hex_lightcovertest (Autodesk Fusion 360 design; units mm, degrees)
Autodesk Fusion 360 part; units mm, degrees
sketch "Sketch1" plane through (0, 12, 0) normal (0, -1, 0) x (1, 0, 0)
  line L0 (-41.8393, 72.4678) -> (-83.6786, 0)
  line L1 (-83.6786, 0) -> (-41.8393, -72.4678)
  line L2 (-41.8393, -72.4678) -> (41.8393, -72.4678)
  line L3 (41.8393, -72.4678) -> (83.6786, 0)
  line L4 (83.6786, 0) -> (41.8393, 72.4678)
  line L5 (41.8393, 72.4678) -> (-41.8393, 72.4678)
  line L6 (-41.8393, 72.4678) -> (41.8393, 72.4678)
  line L7 (41.8393, 72.4678) -> (83.6786, 0)
  line L8 (83.6786, 0) -> (41.8393, -72.4678)
  line L9 (41.8393, -72.4678) -> (-41.8393, -72.4678)
  line L10 (-41.8393, -72.4678) -> (-83.6786, 0)
  line L11 (-83.6786, 0) -> (-41.8393, 72.4678)
  line L12 (82.0621, 0) -> (41.031, -71.0678)
  line L13 (41.031, -71.0678) -> (-41.031, -71.0678)
  line L14 (-41.031, -71.0678) -> (-82.0621, 0)
  line L15 (-82.0621, 0) -> (-41.031, 71.0678)
  line L16 (-41.031, 71.0678) -> (41.031, 71.0678)
  line L17 (41.031, 71.0678) -> (82.0621, 0)
  dimension "d1" = 1.4
  constraint coincident L0.start L5.end
  constraint coincident L4.end L5.start
  constraint coincident L3.end L4.start
  constraint coincident L2.end L3.start
  constraint coincident L1.end L2.start
  constraint coincident L0.end L1.start
sketch "Sketch2" plane through (0, 12, 0) normal (0, 1, 0) x (-1, 0, 0)
  line L0 (-42.4167, 73.4678) -> (42.4167, 73.4678)
  line L1 (42.4167, 73.4678) -> (84.8333, 0)
  line L2 (84.8333, 0) -> (42.4167, -73.4678)
  line L3 (42.4167, -73.4678) -> (-42.4167, -73.4678)
  line L4 (-42.4167, -73.4678) -> (-84.8333, 0)
  line L5 (-84.8333, 0) -> (-42.4167, 73.4678)
  line L6 (-43.5714, 75.4678) -> (-87.1427, 0)
  line L7 (-87.1427, 0) -> (-43.5714, -75.4678)
  line L8 (-43.5714, -75.4678) -> (43.5714, -75.4678)
  line L9 (43.5714, -75.4678) -> (87.1427, 0)
  line L10 (87.1427, 0) -> (43.5714, 75.4678)
  line L11 (43.5714, 75.4678) -> (-43.5714, 75.4678)
  line L12 (-43.5714, 75.4678) -> (43.5714, 75.4678)
  line L13 (87.1427, 0) -> (43.5714, 75.4678)
  line L14 (87.1427, 0) -> (43.5714, -75.4678)
  line L15 (43.5714, -75.4678) -> (-43.5714, -75.4678)
  line L16 (-43.5714, -75.4678) -> (-87.1427, 0)
  line L17 (-87.1427, 0) -> (-43.5714, 75.4678)
  constraint coincident L6.start L11.end
  constraint coincident L10.end L11.start
  constraint coincident L9.end L10.start
  constraint coincident L8.end L9.start
  constraint coincident L7.end L8.start
  constraint coincident L6.end L7.start
sketch "Sketch3" plane through (0, 4, 0) normal (0, 1, 0) x (-1, 0, 0)
  line L0 (-38.9526, -67.4678) -> (-77.9051, 0)
  line L1 (-77.9051, 0) -> (-38.9526, 67.4678)
  line L2 (-38.9526, 67.4678) -> (38.9526, 67.4678)
  line L3 (38.9526, 67.4678) -> (77.9051, 0)
  line L4 (77.9051, 0) -> (38.9526, -67.4678)
  line L5 (38.9526, -67.4678) -> (-38.9526, -67.4678)
  line L6 (-84.8333, 0) -> (-42.4167, -73.4678)
  line L7 (-42.4167, -73.4678) -> (42.4167, -73.4678)
  line L8 (42.4167, -73.4678) -> (84.8333, 0)
  line L9 (84.8333, 0) -> (42.4167, 73.4678)
  line L10 (42.4167, 73.4678) -> (-42.4167, 73.4678)
  line L11 (-42.4167, 73.4678) -> (-84.8333, 0)
  line L12 (42.4167, -73.4678) -> (84.8333, 0)
  line L13 (42.4167, 73.4678) -> (84.8333, 0)
  line L14 (42.4167, 73.4678) -> (-42.4167, 73.4678)
  line L15 (-42.4167, 73.4678) -> (-84.8333, 0)
  line L16 (-84.8333, 0) -> (-42.4167, -73.4678)
  line L17 (-42.4167, -73.4678) -> (42.4167, -73.4678)
  line L18 (-42.4167, 73.4678) -> (-84.8333, 0)
  line L19 (-41.8393, -72.4678) -> (41.8393, -72.4678)
  line L20 (41.8393, -72.4678) -> (83.6786, 0)
  line L21 (41.8393, 72.4678) -> (83.6786, 0)
  line L22 (41.8393, 72.4678) -> (-41.8393, 72.4678)
  line L23 (-41.8393, 72.4678) -> (-83.6786, 0)
  line L24 (-83.6786, 0) -> (-41.8393, -72.4678)
  line L25 (41.031, 71.0678) -> (-41.031, 71.0678)
  line L26 (-41.031, 71.0678) -> (-82.0621, 0)
  line L27 (-82.0621, 0) -> (-41.031, -71.0678)
  line L28 (-41.031, -71.0678) -> (41.031, -71.0678)
  line L29 (41.031, -71.0678) -> (82.0621, 0)
  line L30 (41.031, 71.0678) -> (82.0621, 0)
  dimension "d2" = -1
  dimension "d3" = -2.4
  constraint coincident L7.end L8.start
  constraint coincident L8.end L9.start
  constraint coincident L9.end L10.start
  constraint coincident L10.end L11.start
  constraint coincident L6.start L11.end
  constraint coincident L6.end L7.start
sketch "Sketch4" plane through (0, 13, 0) normal (0, -1, 0) x (1, 0, 0)
  arc A0 (44.7261, 67.4678) -> (36.0658, 72.4678) centre (36.0658, 62.4678) ccw
  line L0 (44.7261, 67.4678) -> (80.7919, 5)
  arc A1 (80.7919, -5) -> (80.7919, 5) centre (72.1316, 0) ccw
  line L1 (80.7919, -5) -> (44.7261, -67.4678)
  arc A2 (36.0658, -72.4678) -> (44.7261, -67.4678) centre (36.0658, -62.4678) ccw
  line L2 (36.0658, -72.4678) -> (-36.0658, -72.4678)
  arc A3 (-44.7261, -67.4678) -> (-36.0658, -72.4678) centre (-36.0658, -62.4678) ccw
  line L3 (-44.7261, -67.4678) -> (-80.7919, -5)
  arc A4 (-80.7919, 5) -> (-80.7919, -5) centre (-72.1316, 0) ccw
  line L4 (-80.7919, 5) -> (-44.7261, 67.4678)
  arc A5 (-36.0658, 72.4678) -> (-44.7261, 67.4678) centre (-36.0658, 62.4678) ccw
  line L5 (-36.0658, 72.4678) -> (36.0658, 72.4678)
  line L6 (42.4167, 73.4678) -> (-42.4167, 73.4678)
  line L7 (-42.4167, 73.4678) -> (-84.8333, 0)
  line L8 (-84.8333, 0) -> (-42.4167, -73.4678)
  line L9 (-42.4167, -73.4678) -> (42.4167, -73.4678)
  line L10 (42.4167, -73.4678) -> (84.8333, 0)
  line L11 (84.8333, 0) -> (42.4167, 73.4678)
  line L12 (-42.4167, 73.4678) -> (-32.4167, 73.4678)
  line L13 (-42.4167, 73.4678) -> (-47.4167, 64.8076)
  line L14 (-32.4167, 73.4678) -> (-32.4167, 56.1473)
  line L15 (-47.4167, 64.8076) -> (-32.4167, 56.1473)
  dimension "d4" = 10
  dimension "d5" = 0
  constraint coincident L6.end L7.start
  constraint coincident L6 L12.end
  constraint parallel L6 L12
  constraint coincident L7 L13.end
  constraint parallel L7 L13
  constraint perpendicular L5 L14
  constraint perpendicular L13 L15
  constraint coincident L14.end L15.end
  measures "d4" distance of L6.end L13.end
  measures "d5" distance of L6.end L12.end
extrude "Extrude1" add sketch "Sketch2" along normal blind 3 contours L0 L1 L2 L3 L4 L5 | L6 L7 L8 L9 L10 L11 L12 L13 L14 L15 L16 L17
extrude "Extrude2" cut sketch "Sketch3" along normal blind -1 and the other way blind -9 contours L6 L7 L8 L9 L10 L11 L12 L13 L14 L15 L16 L17 L18
move_face "OffsetFaces1" [suppressed]
extrude "Extrude3" cut sketch "Sketch1" against normal blind 2.6 contours L12 L13 L14 L15 L16 L17
fillet "Fillet1" radius 10 6 edges at (-83.6786, 12.5, 0) (-41.8393, 12.5, 72.4678) (41.8393, 12.5, 72.4678) (83.6786, 12.5, 0) (41.8393, 12.5, -72.4678) (-41.8393, 12.5, -72.4678)
fillet "Fillet1" radius 10 6 edges at (-41.031, 13.3, 71.0678) (-82.0621, 13.3, 0) (-41.031, 13.3, -71.0678) (41.031, 13.3, -71.0678) (82.0621, 13.3, 0) (41.031, 13.3, 71.0678)
chamfer "Chamfer1" distance 1 angle 45 18 edges at (63.625, 12, 36.7339) (63.625, 12, -36.7339) (82.1316, 12, 0) (62.759, 12, -36.2339) (41.0658, 12, -71.1281) (0, 12, -72.4678) (-41.0658, 12, -71.1281) (-62.759, 12, -36.2339) (-82.1316, 12, 0) (-62.759, 12, 36.2339) (-41.0658, 12, 71.1281) (0, 12, 72.4678) (41.0658, 12, 71.1281) (62.759, 12, 36.2339) (0, 12, 73.4678) (-63.625, 12, 36.7339) (-63.625, 12, -36.7339) (0, 12, -73.4678)
sketch "Sketch5" plane through (0, 14.6, 0) normal (0, -1, 0) x (1, 0, 0)
  arc A0 (43.9178, 66.0678) -> (35.2575, 71.0678) centre (35.2575, 61.0678) ccw
  line L0 (35.2575, 71.0678) -> (-35.2575, 71.0678)
  arc A1 (-35.2575, 71.0678) -> (-43.9178, 66.0678) centre (-35.2575, 61.0678) ccw
  line L1 (-43.9178, 66.0678) -> (-79.1753, 5)
  arc A2 (-79.1753, 5) -> (-79.1753, -5) centre (-70.515, 0) ccw
  line L2 (-79.1753, -5) -> (-43.9178, -66.0678)
  arc A3 (-43.9178, -66.0678) -> (-35.2575, -71.0678) centre (-35.2575, -61.0678) ccw
  line L3 (-35.2575, -71.0678) -> (35.2575, -71.0678)
  arc A4 (35.2575, -71.0678) -> (43.9178, -66.0678) centre (35.2575, -61.0678) ccw
  line L4 (43.9178, -66.0678) -> (79.1753, -5)
  arc A5 (79.1753, -5) -> (79.1753, 5) centre (70.515, 0) ccw
  line L5 (79.1753, 5) -> (43.9178, 66.0678)
  line L6 (0, 0) -> (-80.515, 0)
  line L7 (-40.2575, 69.7281) -> (0, 0)
  line L8 (40.2575, 69.7281) -> (-40.2575, -69.7281)
  line L9 (40.2575, -69.7281) -> (0, 0)
  line L10 (80.515, 0) -> (0, 0)
  constraint coincident L6.start L7.end
  constraint midpoint A2 L6.end
  constraint midpoint A1 L7.start
  constraint midpoint A0 L8.start
  constraint midpoint A3 L8.end
  constraint midpoint A4 L9.start
  constraint midpoint A5 L10.start
extrude "Extrude11" add 1 faces at (2.8868, 14.6, -1.6667) along direction (0, -1, 0) blind 3
extrude "Extrude5" [suppressed]
extrude "Extrude6" [suppressed]
extrude "Extrude7" [suppressed]
extrude "Extrude8" [suppressed]
extrude "Extrude9" [suppressed]
sketch "Sketch6" plane through (0, 12, 0) normal (0, -1, 0) x (1, 0, 0)
  line L0 (-35.2575, 71.0678) -> (35.2575, 71.0678)
  arc A0 (43.9178, 66.0678) -> (35.2575, 71.0678) centre (35.2575, 61.0678) ccw
  line L1 (43.9178, 66.0678) -> (79.1753, 5)
  arc A1 (79.1753, -5) -> (79.1753, 5) centre (70.515, 0) ccw
  line L2 (79.1753, -5) -> (43.9178, -66.0678)
  arc A2 (35.2575, -71.0678) -> (43.9178, -66.0678) centre (35.2575, -61.0678) ccw
  line L3 (35.2575, -71.0678) -> (-35.2575, -71.0678)
  arc A3 (-43.9178, -66.0678) -> (-35.2575, -71.0678) centre (-35.2575, -61.0678) ccw
  line L4 (-43.9178, -66.0678) -> (-79.1753, -5)
  arc A4 (-79.1753, 5) -> (-79.1753, -5) centre (-70.515, 0) ccw
  line L5 (-79.1753, 5) -> (-43.9178, 66.0678)
  line L6 (-43.86, 66.9678) -> (-79.9259, 4.5)
  arc A5 (-79.9259, 4.5) -> (-79.9259, -4.5) centre (-72.1316, 0) ccw
  line L7 (-79.9259, -4.5) -> (-43.86, -66.9678)
  arc A6 (-43.86, -66.9678) -> (-36.0658, -71.4678) centre (-36.0658, -62.4678) ccw
  line L8 (-36.0658, -71.4678) -> (36.0658, -71.4678)
  arc A7 (36.0658, -71.4678) -> (43.86, -66.9678) centre (36.0658, -62.4678) ccw
  line L9 (43.86, -66.9678) -> (79.9259, -4.5)
  arc A8 (79.9259, -4.5) -> (79.9259, 4.5) centre (72.1316, 0) ccw
  line L10 (79.9259, 4.5) -> (43.86, 66.9678)
  arc A9 (43.86, 66.9678) -> (36.0658, 71.4678) centre (36.0658, 62.4678) ccw
  line L11 (36.0658, 71.4678) -> (-36.0658, 71.4678)
  arc A10 (-35.2575, 71.0678) -> (-43.9178, 66.0678) centre (-35.2575, 61.0678) ccw
  arc A11 (-36.0658, 71.4678) -> (-43.86, 66.9678) centre (-36.0658, 62.4678) ccw
  line L12 (-79.1753, 5) -> (-43.9178, 66.0678)
  arc A12 (-35.2575, 71.0678) -> (-43.9178, 66.0678) centre (-35.2575, 61.0678) ccw
  line L13 (-35.2575, 71.0678) -> (35.2575, 71.0678)
  arc A13 (43.9178, 66.0678) -> (35.2575, 71.0678) centre (35.2575, 61.0678) ccw
  line L14 (43.9178, 66.0678) -> (79.1753, 5)
  arc A14 (79.1753, -5) -> (79.1753, 5) centre (70.515, 0) ccw
  line L15 (79.1753, -5) -> (43.9178, -66.0678)
  arc A15 (35.2575, -71.0678) -> (43.9178, -66.0678) centre (35.2575, -61.0678) ccw
  line L16 (35.2575, -71.0678) -> (-35.2575, -71.0678)
  arc A16 (-43.9178, -66.0678) -> (-35.2575, -71.0678) centre (-35.2575, -61.0678) ccw
  line L17 (-43.9178, -66.0678) -> (-79.1753, -5)
  arc A17 (-79.1753, 5) -> (-79.1753, -5) centre (-70.515, 0) ccw
  arc A18 (79.9259, -4.5) -> (79.9259, 4.5) centre (72.1316, 0) ccw
  line L18 (79.9259, 4.5) -> (43.86, 66.9678)
  arc A19 (43.86, 66.9678) -> (36.0658, 71.4678) centre (36.0658, 62.4678) ccw
  line L19 (36.0658, 71.4678) -> (-36.0658, 71.4678)
  arc A20 (-36.0658, 71.4678) -> (-43.86, 66.9678) centre (-36.0658, 62.4678) ccw
  line L20 (-43.86, 66.9678) -> (-79.9259, 4.5)
  arc A21 (-79.9259, 4.5) -> (-79.9259, -4.5) centre (-72.1316, 0) ccw
  line L21 (-79.9259, -4.5) -> (-43.86, -66.9678)
  arc A22 (-43.86, -66.9678) -> (-36.0658, -71.4678) centre (-36.0658, -62.4678) ccw
  line L22 (-36.0658, -71.4678) -> (36.0658, -71.4678)
  arc A23 (36.0658, -71.4678) -> (43.86, -66.9678) centre (36.0658, -62.4678) ccw
  line L23 (43.86, -66.9678) -> (79.9259, -4.5)
  arc A24 (42.8785, 65.4678) -> (35.2575, 69.8678) centre (35.2575, 61.0678) ccw
  line L24 (-35.2575, 69.8678) -> (35.2575, 69.8678)
  arc A25 (-35.2575, 69.8678) -> (-42.8785, 65.4678) centre (-35.2575, 61.0678) ccw
  line L25 (-78.1361, 4.4) -> (-42.8785, 65.4678)
  arc A26 (-78.1361, 4.4) -> (-78.1361, -4.4) centre (-70.515, 0) ccw
  line L26 (-42.8785, -65.4678) -> (-78.1361, -4.4)
  arc A27 (-42.8785, -65.4678) -> (-35.2575, -69.8678) centre (-35.2575, -61.0678) ccw
  line L27 (35.2575, -69.8678) -> (-35.2575, -69.8678)
  arc A28 (35.2575, -69.8678) -> (42.8785, -65.4678) centre (35.2575, -61.0678) ccw
  line L28 (78.1361, -4.4) -> (42.8785, -65.4678)
  arc A29 (78.1361, -4.4) -> (78.1361, 4.4) centre (70.515, 0) ccw
  line L29 (42.8785, 65.4678) -> (78.1361, 4.4)
  arc A30 (-35.2575, 70.0678) -> (-43.0518, 65.5678) centre (-35.2575, 61.0678) ccw
  line L30 (-78.3093, 4.5) -> (-43.0518, 65.5678)
  arc A31 (-78.3093, 4.5) -> (-78.3093, -4.5) centre (-70.515, 0) ccw
  line L31 (-43.0518, -65.5678) -> (-78.3093, -4.5)
  arc A32 (-43.0518, -65.5678) -> (-35.2575, -70.0678) centre (-35.2575, -61.0678) ccw
  line L32 (35.2575, -70.0678) -> (-35.2575, -70.0678)
  arc A33 (35.2575, -70.0678) -> (43.0518, -65.5678) centre (35.2575, -61.0678) ccw
  line L33 (78.3093, -4.5) -> (43.0518, -65.5678)
  arc A34 (78.3093, -4.5) -> (78.3093, 4.5) centre (70.515, 0) ccw
  line L34 (43.0518, 65.5678) -> (78.3093, 4.5)
  arc A35 (43.0518, 65.5678) -> (35.2575, 70.0678) centre (35.2575, 61.0678) ccw
  line L35 (-35.2575, 70.0678) -> (35.2575, 70.0678)
  dimension "d16" = 1.2
  dimension "d17" = 1
extrude "Extrude10" [suppressed]
extrude "Extrude4" [suppressed]
chamfer "Chamfer2" [suppressed]
equation "d5 = d154"
